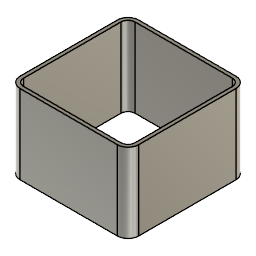
▢-150×150×4.5 (Autodesk Fusion 360 design; units mm, degrees)
Autodesk Fusion 360 part; units mm, degrees
sketch "スケッチ1" plane through (0, 0, 0) normal (0, 0, 1) x (1, 0, 0)
  arc A0 (506.3587, 411.6011) -> (492.8587, 398.1011) centre (506.3587, 398.1011) ccw
  arc A1 (506.3587, 407.1011) -> (497.3587, 398.1011) centre (506.3587, 398.1011) ccw
  arc A2 (642.8587, 398.1011) -> (629.3587, 411.6011) centre (629.3587, 398.1011) ccw
  arc A3 (638.3587, 398.1011) -> (629.3587, 407.1011) centre (629.3587, 398.1011) ccw
  line L0 (506.3587, 261.6011) -> (629.3587, 261.6011)
  line L1 (506.3587, 266.1011) -> (629.3587, 266.1011)
  arc A4 (492.8587, 275.1011) -> (506.3587, 261.6011) centre (506.3587, 275.1011) ccw
  arc A5 (497.3587, 275.1011) -> (506.3587, 266.1011) centre (506.3587, 275.1011) ccw
  line L2 (492.8587, 398.1011) -> (492.8587, 275.1011)
  line L3 (497.3587, 398.1011) -> (497.3587, 275.1011)
  arc A6 (629.3587, 261.6011) -> (642.8587, 275.1011) centre (629.3587, 275.1011) ccw
  arc A7 (629.3587, 266.1011) -> (638.3587, 275.1011) centre (629.3587, 275.1011) ccw
  line L4 (638.3587, 275.1011) -> (638.3587, 398.1011)
  line L5 (642.8587, 275.1011) -> (642.8587, 398.1011)
  line L6 (629.3587, 411.6011) -> (506.3587, 411.6011)
  line L7 (629.3587, 407.1011) -> (506.3587, 407.1011)
  point P0 (567.8587, 336.6011)
extrude "押し出し1" add sketch "スケッチ1" along normal blind 100
